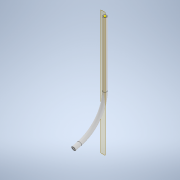
# Autodesk Inventor part: Stainless steel tube
Saved by Autodesk Inventor 2021.2 (Build 252289000, 289)
## iProperties
Created: 2021-06-30
Part Number: Stainless steel tube
Material: Generic
Document SubType Name: Modeling
Designer: jl4459
Density: 1 g/cm^3
Appearance: Default
Author: jl4459
Autodesk Inventor part; units mm, degrees
ref_plane "YZ Plane" through (0, 0, 0) normal (1, 0, 0) x (0, 1, 0)
ref_plane "XZ Plane" through (0, 0, 0) normal (0, 1, 0) x (-1, 0, 0)
sketch "Sketch1" plane through (0, 0, 0) normal (0, 1, 0) x (-1, 0, 0)
  circle A0 centre (0, 0) radius 3.175
  circle A1 centre (0, 0) radius 1.524
  dimension "d0" = 6.35
  dimension "d1" = 3.048
  constraints: 2 centre point, 2 coincident
  measures "d0" diameter of A0
  measures "d1" diameter of A1
extrude "Extrusion1" add sketch "Sketch1" along normal blind 177.8
sketch "Sketch2" plane through (0, 177.8, 0) normal (0, 1, 0) x (1, 0, 0)
  point P0 (0, 0)
sketch "Sketch3" plane through (0, 177.8, 0) normal (0, 1, 0) x (1, 0, 0)
  point P0 (0, 0)
ref_plane "Work Plane1" through (0, 0, 3.175) normal (0, 0, 1) x (1, 0, 0)
sketch "Sketch4" plane through (0, 0, 3.175) normal (0, 0, 1) x (1, 0, 0)
  line L0 (-15.875, 25.4) -> (22.225, 25.4)
  line L1 (-15.8266, 76.2) -> (22.2734, 76.2)
  point P0 (0, 0)
  dimension "d4" = 38.1
  dimension "d5" = 25.4
  dimension "d6" = 38.1
  dimension "d7" = 76.2
  constraints: 4 end point, 2 horizontal
  measures "d4" distance of L0.start L0.end
  measures "d5" distance from line of L0 point (0, 0)
  measures "d6" distance of L1.start L1.end
  measures "d7" distance from line of L1 point (0, 0)
bend part "Bend Part1" radius 50.8 angle 75 line through (-15.8266, 76.2, 3.175) along (1, 0, 0) centre toward (0, 0, 1) moving side (0, -1, 0) both sides no
hole "Hole1" at (0, 177.8, 0) direction (0, -1, 0) diameter 3.9624 depth 6.35 thread size "10-32 UNF" class "2B" standard "ANSI Unified Screw Threads"
sketch "Sketch8" plane through (0, 21.5528, 49.3776) normal (0, -0.258819, 0.9659258) x (1, 0, 0)
  circle A0 centre (0, 0) radius 3.175 projected
  circle A1 centre (0, 0) radius 1.524
  point P0 (0, -33.5983)
  constraints: 1 centre point, 1 coincident
hole "Hole4" at (0, 21.5528, 49.3776) direction (0, 0.258819, -0.9659258) diameter 3.9624 depth 6.35 thread size "10-32 UNF" class "2B" standard "ANSI Unified Screw Threads"
body "Solid1"
